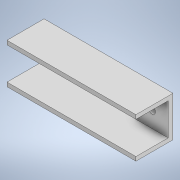
# Autodesk Inventor part: Verbinder
Saved by Autodesk Inventor 2021 (Build 250183000, 183)
## iProperties
Created: 2024-02-03
Part Number: Verbinder
Material: Generic
Document SubType Name: Modeling
Designer: Lukas
Density: 1 g/cm^3
Appearance: Default
Author: Lukas
Autodesk Inventor part; units mm, degrees
ref_plane "YZ Plane" through (0, 0, 0) normal (1, 0, 0) x (0, 1, 0)
ref_plane "XZ Plane" through (0, 0, 0) normal (0, 1, 0) x (-1, 0, 0)
ref_plane "XY Plane" through (0, 0, 0) normal (0, 0, 1) x (1, 0, 0)
sketch "Sketch1" plane through (0, 0, 0) normal (0, 0, 1) x (1, 0, 0)
  line L0 (-40, 12.5) -> (40, 12.5)
  line L1 (40, 12.5) -> (40, -12.5)
  line L2 (40, -12.5) -> (-40, -12.5)
  line L3 (-40, -12.5) -> (-40, 12.5)
  circle A0 centre (-30, 0) radius 2.15
  circle A1 centre (-5, 0) radius 2.15
  circle A2 centre (5, 0) radius 2.15
  circle A3 centre (30, 0) radius 2.15
  point P0 (0, 0)
  point P1 (0, 12.5)
  point P2 (-40, 0)
  dimension "d0" = 25
  dimension "d1" = 80
  dimension "d9" = 4.3
  dimension "d10" = 5
  dimension "d11" = 5
  dimension "d12" = 10
  dimension "d13" = 10
  constraints: 8 end point, 5 horizontal alignment, 4 centre point, 3 equal radius, 2 midpoint, 2 parallel, 1 horizontal, 1 perpendicular, 1 vertical alignment
  measures "d0" distance of L2.end L0.start
  measures "d1" distance of L0.start L0.end
  measures "d9" diameter of A0
  measures "d10" distance of point (0, 0) A1.centre
  measures "d11" distance of point (0, 0) A2.centre
  measures "d12" distance from line of L1 A3.centre
  measures "d13" distance from line of L3 A0.centre
extrude "Extrusion1" add sketch "Sketch1" along normal blind 3
sketch "Sketch2" plane through (0, 0, 3) normal (0, 0, 1) x (1, 0, 0)
  line L0 (-40, -12.5) -> (40, -12.5) projected
  line L1 (40, -12.5) -> (40, 12.5) projected
  line L2 (40, 12.5) -> (-40, 12.5) projected
  line L3 (-40, 12.5) -> (-40, -12.5) projected
  line L4 (-40, 12.5) -> (-40, -12.5) projected
  line L5 (-40, 10) -> (40, 10)
  line L6 (40, -12.5) -> (40, 12.5) projected
  line L7 (40, -12.5) -> (40, 12.5) projected
  line L8 (40, -10) -> (-40, -10)
  point P0 (0, 0)
  dimension "d4" = 2.5
  dimension "d5" = 2.5
  dimension "d6" = 20
  constraints: 4 end point, 4 point on line, 1 horizontal, 1 perpendicular
  measures "d4" distance between parallel lines of L2 L5
  measures "d5" distance between parallel lines of L0 L8
  measures "d6" distance between parallel lines of L5 L8
extrude "Extrusion2" add sketch "Sketch2" along normal blind 20 contours L3 L8 L1 L0 | L3 L2 L1 L5
equation "\"d11\" = d10"
equation "\"d12\" = 2 * d10"
equation "\"d13\" = d12"
equation "\"d5\" = d4"
body "Solid1"
